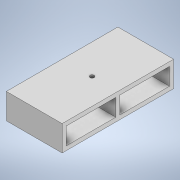
# Autodesk Inventor part: Lenkung
Saved by Autodesk Inventor 2020.3 (Build 243373010, 373A)
## iProperties
Created: 2020-11-21
Part Number: Lenkung
Material: Generisch
Document SubType Name: Modeling
Designer: Stefan
Density: 1 g/cm^3
Appearance: Vorgabe
Author: Stefan
Autodesk Inventor part; units mm, degrees
ref_plane "YZ Plane" through (0, 0, 0) normal (1, 0, 0) x (0, 1, 0)
ref_plane "XZ Plane" through (0, 0, 0) normal (0, 1, 0) x (-1, 0, 0)
ref_plane "XY Plane" through (0, 0, 0) normal (0, 0, 1) x (1, 0, 0)
sketch "Skizze2" plane through (0, 0, 0) normal (0, 1, 0) x (-1, 0, 0)
  line L0 (75, 150) -> (-75, 150)
  line L1 (-75, 150) -> (-75, -150)
  line L2 (-75, -150) -> (75, -150)
  line L3 (75, -150) -> (75, 150)
  point P0 (0, 0)
  dimension "d4" = 150
  dimension "d5" = 300
  dimension "d6" = 150
  dimension "d7" = 75
  constraints: 8 end point, 2 parallel, 1 horizontal, 1 perpendicular
  measures "d4" distance of L2.end L1.end
  measures "d5" distance of L2.end L0.start
  measures "d6" distance from line of point (0, 0) L2
  measures "d7" distance from line of L1 point (0, 0)
extrude "Extrusion2" add sketch "Skizze2" along normal blind 12
sketch "Skizze3" plane through (-75, 0, -150) normal (-1, 0, 0) x (0, 0, 1)
  line L0 (300, 0) -> (0, 0) projected
  line L1 (0, 0) -> (300, 0)
  line L2 (300, 0) -> (300, 74)
  line L3 (300, 74) -> (0, 74)
  line L4 (0, 74) -> (0, 0)
  point P0 (150, 0)
  dimension "d10" = 300
  dimension "d11" = 74
  constraints: 8 end point, 2 parallel, 1 horizontal, 1 perpendicular
  measures "d10" distance of L3.end L2.end
  measures "d11" distance of L2.end L1.end
extrude "Extrusion3" add sketch "Skizze3" along normal blind 12
sketch "Skizze4" plane through (-75, 0, -150) normal (1, 0, 0) x (0, 0, -1)
  line L0 (-300, 12) -> (-300, 74) projected
  line L1 (-300, 74) -> (0, 74)
  line L2 (0, 74) -> (0, 62)
  line L3 (0, 62) -> (-300, 62)
  line L4 (-300, 62) -> (-300, 74)
  point P0 (-150, 0)
  dimension "d14" = 300
  dimension "d15" = 12
  constraints: 8 end point, 2 parallel, 1 horizontal, 1 perpendicular
  measures "d14" distance of L2.end L3.end
  measures "d15" distance of L1.end L2.end
extrude "Extrusion4" add sketch "Skizze4" along normal blind 150
sketch "Skizze5" plane through (75, 0, 150) normal (0, 0, 1) x (1, 0, 0)
  line L0 (0, 0) -> (-162, 0) projected
  line L1 (0, 62) -> (0, 74) projected
  line L2 (-162, 0) -> (0, 0)
  line L3 (0, 0) -> (0, 74)
  line L4 (0, 74) -> (-162, 74)
  line L5 (-162, 74) -> (-162, 0)
  point P0 (-75, 0)
  constraints: 8 end point, 2 parallel, 1 horizontal, 1 perpendicular
extrude "Extrusion5" add sketch "Skizze5" along normal blind 12
sketch "Skizze6" plane through (75, 0, -150) normal (0, 0, -1) x (-1, 0, 0)
  line L0 (0, 0) -> (0, 12) projected
  line L1 (162, 74) -> (162, 0) projected
  line L2 (0, 0) -> (162, 0)
  line L3 (162, 0) -> (162, 74)
  line L4 (162, 74) -> (0, 74)
  line L5 (0, 74) -> (0, 0)
  point P0 (75, 0)
  point P1 (162, 0)
  constraints: 8 end point, 2 parallel, 1 horizontal, 1 perpendicular
extrude "Extrusion6" add sketch "Skizze6" along normal blind 12
sketch "Skizze7" plane through (-87, 74, 162) normal (0, 1, 0) x (1, 0, 0)
  point P0 (87, 162)
hole "Bohrung1" at (0, 74, 0) direction (0, -1, 0) diameter 12 end through all
sketch "Skizze8" plane through (-75, 0, -150) normal (1, 0, 0) x (0, 0, -1)
  line L0 (0, 62) -> (-300, 62) projected
  line L1 (0, 12) -> (-300, 12) projected
  line L2 (-156, 62) -> (-144, 62)
  line L3 (-144, 62) -> (-144, 12)
  line L4 (-144, 12) -> (-156, 12)
  line L5 (-156, 12) -> (-156, 62)
  line L6 (0, 62) -> (0, 12) projected
  point P0 (-150, 0)
  dimension "d29" = 12
  dimension "d30" = 144
  constraints: 8 end point, 2 parallel, 2 point on line, 1 horizontal, 1 perpendicular
  measures "d29" distance between parallel lines of L3 L5
  measures "d30" distance between parallel lines of L6 L3
extrude "Extrusion7" add sketch "Skizze8" along normal blind 65 contours L3 L1 L5 L0
sketch "Skizze9" plane through (-10, 0, -150) normal (1, 0, 0) x (0, 0, -1)
  point P0 (-150, 0)
fillet "Rundung1" radius 4 2 edges at (-10, 37, 6) (-10, 37, -6)
sketch "Skizze11" plane through (75, 0, 162) normal (1, 0, 0) x (0, 0, -1)
  line L0 (12, 12) -> (312, 12) projected
  line L1 (156, 12) -> (168, 12)
  line L2 (168, 12) -> (168, 62)
  line L3 (168, 62) -> (156, 62)
  line L4 (156, 62) -> (156, 12)
  line L5 (156, 12) -> (156, 62) projected
  point P0 (162, 0)
  dimension "d36" = 12
  dimension "d37" = 50
  dimension "d38" = 0
  constraints: 8 end point, 2 parallel, 1 horizontal, 1 perpendicular, 1 point on line
  measures "d36" distance of L3.end L2.end
  measures "d37" distance of L2.end L1.end
  measures "d38" distance between parallel lines of L5 L4
extrude "Extrusion9" add sketch "Skizze11" against normal blind 65
fillet "Rundung2" radius 4 2 edges at (10, 37, 6) (10, 37, -6)
sketch "Skizze12" plane through (75, 0, 162) normal (1, 0, 0) x (0, 0, -1)
  line L0 (324, 74) -> (0, 74) projected
  line L1 (0, 74) -> (324, 74)
  line L2 (324, 74) -> (324, 0)
  line L3 (324, 0) -> (0, 0)
  line L4 (0, 0) -> (0, 74)
  point P0 (162, 0)
  constraints: 8 end point, 2 parallel, 1 horizontal, 1 perpendicular
extrude "Extrusion10" [suppressed]
